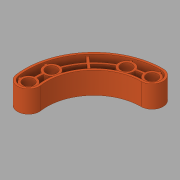
# Autodesk Inventor part: Curved_beam_6h-05
Saved by Autodesk Inventor 2019.3 (Build 233278000, 278)
## iProperties
Created: 2019-01-29
Part Number: Curved_beam_6h-05
Material: Generic
Document SubType Name: Modeling
Designer: Varga Daniel
Density: 1 g/cm^3
Appearance: Copper - 7579 C
Inner_diameter: 43,000 mm
End_hole_dist: 40,000 mm
Author: Varga Daniel
Autodesk Inventor part; units mm, degrees
ref_plane "YZ Plane" through (0, 0, 0) normal (1, 0, 0) x (0, 1, 0)
ref_plane "XZ Plane" through (0, 0, 0) normal (0, 1, 0) x (-1, 0, 0)
ref_plane "XY Plane" through (0, 0, 0) normal (0, 0, 1) x (1, 0, 0)
derived "Base_part.ipt"
sketch "Beam_sketch" plane through (0, 0, 0) normal (0, 1, 0) x (-1, 0, 0)
  line L0 (5, 0) -> (25, 0)
  line L1 (30, 5) -> (30, 25)
  line L2 (25, 30) -> (5, 30)
  line L3 (0, 25) -> (0, 5)
  line L4 (5, 29) -> (25, 29)
  line L5 (29, 25) -> (29, 5)
  line L6 (25, 1) -> (5, 1)
  line L7 (1, 5) -> (1, 25)
  circle A0 centre (5, 5) radius 2.5
  circle A1 centre (5, 5) radius 3.5
  arc A2 (25, 0) -> (30, 5) centre (25, 5) ccw
  arc A3 (30, 25) -> (25, 30) centre (25, 25) ccw
  arc A4 (5, 30) -> (0, 25) centre (5, 25) ccw
  arc A5 (0, 5) -> (5, 0) centre (5, 5) ccw
  arc A6 (1, 5) -> (5, 1) centre (5, 5) ccw
  arc A7 (5, 29) -> (1, 25) centre (5, 25) ccw
  arc A8 (29, 25) -> (25, 29) centre (25, 25) ccw
  arc A9 (25, 1) -> (29, 5) centre (25, 5) ccw
  line L8 (49.1041, 15) -> (-27.081, 15) construction
  circle A10 centre (15, 5) radius 2.5
  circle A11 centre (15, 5) radius 3.5
  line L9 (31.1478, 10) -> (-2.4877, 10) construction
  line L10 (-2.8604, 5) -> (35.495, 5) construction
  line L11 (5, -2.5736) -> (5, 36.7522) construction
  line L12 (15, -1.4978) -> (15, 34.8784) construction
  line L13 (18.4641, 5.5) -> (21.5359, 5.5)
  line L14 (18.4641, 4.5) -> (21.5359, 4.5)
  line L15 (1.5359, 5.5) -> (1, 5.5)
  line L16 (1.5359, 4.5) -> (1.0314, 4.5)
  line L17 (28.9686, 4.5) -> (8.4641, 4.5)
  line L18 (29, 5.5) -> (8.4641, 5.5)
  line L19 (4.5, 1.5359) -> (4.5, 1.0314)
  line L20 (5.5, 1.5359) -> (5.5, 1)
  line L21 (29, 10.5) -> (1, 10.5)
  line L22 (29, 9.5) -> (1, 9.5)
  line L23 (4.5, 28.9686) -> (4.5, 10.5)
  line L24 (4.5, 9.5) -> (4.5, 8.4641)
  line L25 (5.5, 29) -> (5.5, 10.5)
  line L26 (5.5, 9.5) -> (5.5, 8.4641)
  point P0 (0, 0)
  point P1 (30, 30)
  point P2 (0, 30)
sketch "Sketch2" plane through (0, 0, 0) normal (0, 1, 0) x (-1, 0, 0)
  arc A0 (0, -21.5) -> (21.2907, 2.9927) centre (0, 0) ccw
  arc A1 (0, -26.5) -> (26.242, 3.6887) centre (0, 0) ccw construction
  arc A2 (0, -31.5) -> (31.1933, 4.3847) centre (0, 0) ccw
  line L0 (0, -21.5) -> (0, -31.5) construction
  line L1 (21.2907, 2.9927) -> (31.1933, 4.3847) construction
  arc A3 (0, -22.5) -> (22.281, 3.1319) centre (0, 0) ccw
  arc A4 (0, -30.5) -> (30.2031, 4.2455) centre (0, 0) ccw
  circle A5 centre (0, -26.5) radius 3.5
  circle A6 centre (9.8204, -24.6132) radius 3.5
  arc A7 (0, -21.5) -> (0, -31.5) centre (0, -26.5) ccw
  arc A8 (0, -22.5) -> (0, -30.5) centre (0, -26.5) ccw
  arc A9 (31.1933, 4.3847) -> (21.2907, 2.9927) centre (26.242, 3.6887) ccw
  arc A10 (30.2031, 4.2455) -> (22.281, 3.1319) centre (26.242, 3.6887) ccw
  circle A11 centre (26.242, 3.6887) radius 3.5
  circle A12 centre (25.7405, -6.2987) radius 3.5
  line L2 (0, 0) -> (23.7736, -20.6656) construction
  arc A13 (26.0272, 7.1821) -> (25.8868, 7.6729) centre (0, 0) ccw
  arc A14 (25.0461, 6.978) -> (24.907, 7.4593) centre (0, 0) ccw
  arc A15 (25.8487, -2.8004) -> (25.9993, 0.1971) centre (0, 0) ccw
  arc A16 (26.8357, -2.9745) -> (26.9986, 0.2714) centre (0, 0) ccw
  arc A17 (12.7312, -22.6697) -> (24.2212, -9.4517) centre (0, 0) ccw
  arc A18 (13.1626, -23.5742) -> (25.1769, -9.7531) centre (0, 0) ccw
  arc A19 (-3.9198, -25.7028) -> (-3.4238, -25.7736) centre (0, 0) ccw
  arc A20 (3.4238, -25.7736) -> (6.3712, -25.2073) centre (0, 0) ccw
  arc A21 (-3.9949, -26.7028) -> (-3.4893, -26.7736) centre (0, 0) ccw
  arc A22 (3.4893, -26.7736) -> (6.6809, -26.1604) centre (0, 0) ccw
  line L3 (0, -26.5) -> (0, 0) construction
  line L4 (9.8204, -24.6132) -> (0, 0) construction
  line L5 (25.7405, -6.2987) -> (0, 0) construction
  line L6 (26.242, 3.6887) -> (0, 0) construction
  line L7 (7.8716, -21.0781) -> (8.0723, -21.581)
  line L8 (10.6397, -28.016) -> (10.8368, -28.5099)
  line L9 (8.8004, -20.7076) -> (9.0011, -21.2105)
  line L10 (11.5685, -27.6454) -> (11.7656, -28.1393)
  line L11 (0.5, -22.4944) -> (0.5, -23.0359)
  line L12 (0.5, -29.9641) -> (0.5, -30.4959)
  line L13 (-0.5, -30.4686) -> (-0.5, -29.9641)
  line L14 (-0.5, -23.0359) -> (-0.5, -22.5314)
  circle A23 centre (0, -26.5) radius 2.5
  circle A24 centre (9.8204, -24.6132) radius 2.5
  circle A25 centre (25.7405, -6.2987) radius 2.5
  circle A26 centre (26.242, 3.6887) radius 2.5
  line L15 (21.7309, -5.8323) -> (22.2569, -5.961)
  line L16 (28.9865, -7.6078) -> (29.5031, -7.7342)
  line L17 (21.9686, -4.861) -> (22.4946, -4.9897)
  line L18 (29.2242, -6.6364) -> (29.7408, -6.7628)
  line L19 (30.1024, 4.7362) -> (29.6028, 4.666)
  line L20 (22.742, 3.7016) -> (22.2424, 3.6314)
  line L21 (22.3451, 2.636) -> (22.8812, 2.7114)
  line L22 (29.742, 3.6757) -> (30.2686, 3.7498)
  circle A27 centre (5, 5) radius 2.5 construction
  circle A28 centre (5, 5) radius 3.5 construction
  line L23 (16.6489, -15.1348) -> (19.291, -17.4315)
  line L24 (19.947, -16.6768) -> (17.305, -14.3801)
  line L25 (20.0458, -18.0877) -> (22.6877, -20.3842)
  line L26 (23.3438, -19.6295) -> (20.7019, -17.333)
  dimension "d84" = 7
  dimension "d85" = 7
  dimension "d86" = 7
  dimension "d87" = 7
  dimension "d0" = 21.5
  dimension "d5" = 1
  dimension "d14" = 10
  dimension "d15" = 4
  dimension "d21" = 10
  dimension "d34" = 1
  dimension "d35" = 0.5
  dimension "d37" = 1
  dimension "d38" = 1
  dimension "d45" = 5
  dimension "d51" = 1
  dimension "d53" = 1
  dimension "d77" = 4
  dimension "d78" = 4
  dimension "d79" = 5
  dimension "d80" = 7
  dimension "d81" = 5
  dimension "d82" = 5
  dimension "d83" = 5
  dimension "d88" = 1
  dimension "d89" = 40
  constraints: 54 end point, 51 point on circle, 21 centre point, 17 parallel, 12 coincident, 10 collinear, 8 concentric, 7 point on line, 3 midpoint, 2 vertical, 1 tangent, 74 other
  measures "d0" radius of A0
  measures "d14" distance of A1.start L4.start
  measures "d15" radius of A8
  measures "d21" distance of A9.centre L5.start
  measures "d34" radial gap between concentric circles of A20 A22
  measures "d35" radial gap between concentric circles of A1 A22
  measures "d37" distance between parallel lines of L14 L11
  measures "d38" distance between parallel lines of L7 L9
  measures "d45" diameter of A25
  measures "d51" distance between parallel lines of L17 L15
  measures "d53" distance between parallel lines of L20 L21
  measures "d79" diameter of A27
  measures "d80" diameter of A28
  measures "d81" diameter of A23
  measures "d82" diameter of A24
  measures "d83" diameter of A26
  measures "d88" distance between parallel lines of L24 L23
  measures "d89" distance of A1.end A1.start
extrude "Extrusion7" add sketch "Sketch2" along normal mid plane 8.4 contours A3 L11 A5 L14 A8 | A3 L9 A6 L7 | A5 | A19 A5 A21 A8 | A6 | A20 A6 A22 A5 | A3 L24 A17 L23 | L13 A5 L12 A4 A8 | A17 A12 A18 A6 | A3 L17 A12 L15 | A6 L10 A4 L8 | A12 | A18 L26 A4 L25 | A3 A10 L20 A11 L21 | A11 | A15 A11 A16 A12 | A12 L18 A4 L16 | A10 A13 A11 A14 | A11 L19 A10 A4 L22
extrude "Extrusion8" add sketch "Sketch2" along normal mid plane 1 contours A3 L7 A6 A20 A5 L11 | L14 A5 A19 A8 | A3 L23 A17 A6 L9 | A21 A5 L13 A8 | A3 L15 A12 A17 L24 | A6 L8 A4 L12 A5 A22 | A18 L25 A4 L10 A6 | A3 L21 A11 A15 A12 L17 | A12 L16 A4 L26 A18 | A10 A14 A11 L20 | A16 A11 L22 A4 L18 A12 | A10 L19 A11 A13
extrude "Extrusion9" add sketch "Sketch2" along normal mid plane 10 contours A0 A9 A2 A7
equation "\"d5\" = Wall_thickness"
equation "\"d34\" = Inner_route_thickness"
equation "\"d35\" = 0.5 * d34"
equation "\"d37\" = Inner_route_thickness"
equation "\"d38\" = d37"
equation "\"d30\" = Inner_route_thickness"
equation "\"d31\" = 0.5 * d30"
equation "\"d32\" = Inner_route_thickness"
equation "\"d33\" = 0.5 * d32"
equation "\"d39\" = d40"
equation "\"d47\" = d37"
equation "\"Inner_diameter\" = 43"
equation "\"End_hole_dist\" = 40"
equation "\"Wall_thickness\" = 1"
equation "\"Inner_route_thickness\" = 1"
equation "\"d40\" = 5"
body "Solid2"
